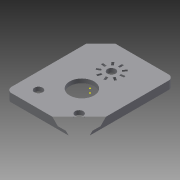
# Autodesk Inventor part: luz
Saved by Autodesk Inventor 2015 SP1 (Build 190203100, 203)
## iProperties
Created: 2015-07-05
Part Number: luz
Material: Genérico
Document SubType Name: Modeling
Designer: Javier
Density: 1 g/cm^3
Appearance: Valor por defecto
Author: Javier
Autodesk Inventor part; units mm, degrees
ref_plane "YZ Plane" through (0, 0, 0) normal (1, 0, 0) x (0, 1, 0)
ref_plane "XZ Plane" through (0, 0, 0) normal (0, 1, 0) x (-1, 0, 0)
ref_plane "XY Plane" through (0, 0, 0) normal (0, 0, 1) x (1, 0, 0)
sketch "Boceto1" plane through (0, 0, 0) normal (0, 0, 1) x (1, 0, 0)
  point P0 (0, 0)
sketch "Boceto2" plane through (0, 0, 0) normal (0, 0, 1) x (1, 0, 0)
  arc A0 (11.5, 13.5) -> (9.5, 15.5) centre (9.5, 13.5) ccw projected
  line L0 (9.5, 15.5) -> (-9.5, 15.5) projected
  arc A1 (-9.5, 15.5) -> (-11.5, 13.5) centre (-9.5, 13.5) ccw projected
  line L1 (-11.5, 13.5) -> (-11.5, -13.5) projected
  arc A2 (-11.5, -13.5) -> (-9.5, -15.5) centre (-9.5, -13.5) ccw projected
  line L2 (-9.5, -15.5) -> (9.5, -15.5) projected
  arc A3 (9.5, -15.5) -> (11.5, -13.5) centre (9.5, -13.5) ccw projected
  line L3 (11.5, -13.5) -> (11.5, 13.5) projected
  circle A4 centre (7.5, -11.5) radius 1.5 projected
  circle A5 centre (-7.5, -11.5) radius 1.5 projected
  line L4 (-4.5, 17.5) -> (-11.5, 17.5) projected
  arc A6 (-11.5, 17.5) -> (-13.5, 15.5) centre (-11.5, 15.5) ccw projected
  line L5 (-13.5, 15.5) -> (-13.5, -15.5) projected
  arc A7 (-13.5, -15.5) -> (-12.3012, -17.3325) centre (-11.5, -15.5) ccw projected
  arc A8 (-11.9943, -17.5) -> (-12.3012, -17.3325) centre (-13.1023, -19.165) ccw projected
  line L6 (11.9943, -17.5) -> (-11.9943, -17.5) projected
  arc A9 (12.3012, -17.3325) -> (11.9943, -17.5) centre (13.1023, -19.165) ccw projected
  arc A10 (12.3012, -17.3325) -> (13.5, -15.5) centre (11.5, -15.5) ccw projected
  line L7 (13.5, -15.5) -> (13.5, 15.5) projected
  arc A11 (13.5, 15.5) -> (11.5, 17.5) centre (11.5, 15.5) ccw projected
  line L8 (11.5, 17.5) -> (4.5, 17.5) projected
  line L9 (-4.5, 16.5) -> (-4.5, 17.5) projected
  line L10 (4.5, 17.5) -> (4.5, 16.5) projected
  line L11 (4.5, 16.5) -> (9.5, 16.5) projected
  arc A12 (12.5, 13.5) -> (9.5, 16.5) centre (9.5, 13.5) ccw projected
  line L12 (12.5, 13.5) -> (12.5, -13.5) projected
  arc A13 (9.5, -16.5) -> (12.5, -13.5) centre (9.5, -13.5) ccw projected
  line L13 (9.5, -16.5) -> (-9.5, -16.5) projected
  arc A14 (-12.5, -13.5) -> (-9.5, -16.5) centre (-9.5, -13.5) ccw projected
  line L14 (-12.5, -13.5) -> (-12.5, 13.5) projected
  arc A15 (-9.5, 16.5) -> (-12.5, 13.5) centre (-9.5, 13.5) ccw projected
  line L15 (-9.5, 16.5) -> (-4.5, 16.5) projected
  circle A16 centre (0, -6) radius 5.5 projected
  line L16 (-4.5, 15.5) -> (-4.5, 17.5)
  line L17 (4.5, 15.5) -> (4.5, 17.5)
  point P0 (0, 0)
  constraints: 4 end point, 2 point on line, 1 parallel, 1 vertical
extrude "Extrusión1" add sketch "Boceto2" along normal blind 2.5 contours A0 L0 L17 L11 A12 L12 A13 L13 A14 L14 A15 L15 L16 A1 L1 A2 L2 A3 L3 | L10 L8 A11 L7 A10 A9 L6 A8 A7 L5 A6 L4 L9 L15 A15 L14 A14 L13 A13 L12 A12 L11
sketch "Boceto3" plane through (0, 0, 2.5) normal (0, 0, 1) x (1, 0, 0)
  point P0 (0, 0)
lip "Labio1" kind lip height 1 width 1 edges at (11.5, 0, 0) (10.9142, -14.9142, 0) (0, -15.5, 0) (-10.9142, -14.9142, 0) (-11.5, 0, 0) (-10.9142, 14.9142, 0) (-7, 15.5, 0) (10.9142, 14.9142, 0) (7, 15.5, 0) guide face at (-12.8333, -4.5, 0)
sketch "Boceto4" plane through (0, 0, 2.5) normal (0, 0, 1) x (1, 0, 0)
  line L0 (-4.5, 17.5) -> (-11.5, 17.5) projected
  arc A0 (-11.5, 17.5) -> (-13.5, 15.5) centre (-11.5, 15.5) ccw projected
  line L1 (-13.5, 15.5) -> (-13.5, -15.5) projected
  arc A1 (-13.5, -15.5) -> (-12.3012, -17.3325) centre (-11.5, -15.5) ccw projected
  line L2 (-11.9943, -17.5) -> (11.9943, -17.5) projected
  arc A2 (12.3012, -17.3325) -> (13.5, -15.5) centre (11.5, -15.5) ccw projected
  line L3 (13.5, -15.5) -> (13.5, 15.5) projected
  arc A3 (13.5, 15.5) -> (11.5, 17.5) centre (11.5, 15.5) ccw projected
  line L4 (11.5, 17.5) -> (4.5, 17.5) projected
  line L5 (-4.5, 17.5) -> (4.5, 17.5)
  circle A4 centre (-7.5, -11.5) radius 1.5 projected
  circle A5 centre (7.5, -11.5) radius 1.5 projected
  line L6 (0, -15.5) -> (0, -3)
  circle A6 centre (0, -3) radius 4.5
  line L7 (12.3062, -17.3254) -> (11.9943, -17.5)
  arc A7 (12.3012, -17.3325) -> (11.9943, -17.5) centre (13.1023, -19.165) ccw projected
  line L8 (-12.3012, -17.3325) -> (-11.9943, -17.5)
  arc A8 (-11.9943, -17.5) -> (-12.3012, -17.3325) centre (-13.1023, -19.165) ccw projected
  dimension "d8" = 12.5
  dimension "d9" = 9
  constraints: 8 end point, 5 centre point, 1 coincident, 1 collinear, 1 vertical
  measures "d8" distance of L6.start L6.end
  measures "d9" diameter of A6
extrude "Extrusión2" add sketch "Boceto4" along normal blind 1.5 contours L5 L4 A3 L3 A2 A7 L2 A8 A1 L1 A0 L0
sketch "Boceto7" plane through (0, 0, 4) normal (0, 0, 1) x (1, 0, 0)
  circle A0 centre (0, -3) radius 4.5 projected
  circle A1 centre (7.5, -11.5) radius 1.5 projected
  circle A2 centre (-7.5, -11.5) radius 1.5 projected
  line L0 (11.5, 17.5) -> (-11.5, 17.5) projected
  arc A3 (-11.5, 17.5) -> (-13.5, 15.5) centre (-11.5, 15.5) ccw projected
  line L1 (-13.5, 15.5) -> (-13.5, -15.5) projected
  arc A4 (-13.5, -15.5) -> (-12.3012, -17.3325) centre (-11.5, -15.5) ccw projected
  line L2 (-11.9943, -17.5) -> (11.9943, -17.5) projected
  arc A5 (12.3012, -17.3325) -> (13.5, -15.5) centre (11.5, -15.5) ccw projected
  line L3 (13.5, -15.5) -> (13.5, 15.5) projected
  arc A6 (13.5, 15.5) -> (11.5, 17.5) centre (11.5, 15.5) ccw projected
  circle A7 centre (0, 7.9359) radius 1.5
  line L4 (-0.375, 12.1766) -> (0.375, 12.1766)
  line L5 (0.375, 12.1766) -> (0.375, 10.6766)
  line L6 (0.375, 10.6766) -> (-0.375, 10.6766)
  line L7 (-0.375, 10.6766) -> (-0.375, 12.1766)
  line L8 (-0.375, 12.1766) -> (0.375, 10.6766) construction
  line L9 (0.375, 12.1766) -> (-0.375, 10.6766) construction
  arc A8 (-11.9943, -17.5) -> (-12.3012, -17.3325) centre (-13.1023, -19.165) ccw projected
  arc A9 (12.3012, -17.3325) -> (11.9943, -17.5) centre (13.1023, -19.165) ccw projected
  line L10 (-3.0131, 10.9434) -> (-2.4386, 11.4255)
  line L11 (-2.4386, 11.4255) -> (-1.4744, 10.2764)
  line L12 (-1.4744, 10.2764) -> (-2.0489, 9.7943)
  line L13 (-2.0489, 9.7943) -> (-3.0131, 10.9434)
  line L14 (-3.0131, 10.9434) -> (-1.4744, 10.2764) construction
  line L15 (-2.4386, 11.4255) -> (-2.0489, 9.7943) construction
  line L16 (-4.2413, 8.303) -> (-4.1111, 9.0416)
  line L17 (-4.1111, 9.0416) -> (-2.6339, 8.7812)
  line L18 (-2.6339, 8.7812) -> (-2.7641, 8.0425)
  line L19 (-2.7641, 8.0425) -> (-4.2413, 8.303)
  line L20 (-4.2413, 8.303) -> (-2.6339, 8.7812) construction
  line L21 (-4.1111, 9.0416) -> (-2.7641, 8.0425) construction
  line L22 (-3.485, 5.4909) -> (-3.86, 6.1404)
  line L23 (-3.86, 6.1404) -> (-2.561, 6.8904)
  line L24 (-2.561, 6.8904) -> (-2.186, 6.2409)
  line L25 (-2.186, 6.2409) -> (-3.485, 5.4909)
  line L26 (-3.485, 5.4909) -> (-2.561, 6.8904) construction
  line L27 (-3.86, 6.1404) -> (-2.186, 6.2409) construction
  line L28 (-1.098, 3.8228) -> (-1.8028, 4.0793)
  line L29 (-1.8028, 4.0793) -> (-1.2897, 5.4888)
  line L30 (-1.2897, 5.4888) -> (-0.585, 5.2323)
  line L31 (-0.585, 5.2323) -> (-1.098, 3.8228)
  line L32 (-1.098, 3.8228) -> (-1.2897, 5.4888) construction
  line L33 (-1.8028, 4.0793) -> (-0.585, 5.2323) construction
  line L34 (1.8028, 4.0793) -> (1.098, 3.8228)
  line L35 (1.098, 3.8228) -> (0.585, 5.2323)
  line L36 (0.585, 5.2323) -> (1.2897, 5.4888)
  line L37 (1.2897, 5.4888) -> (1.8028, 4.0793)
  line L38 (1.8028, 4.0793) -> (0.585, 5.2323) construction
  line L39 (1.098, 3.8228) -> (1.2897, 5.4888) construction
  line L40 (3.86, 6.1404) -> (3.485, 5.4909)
  line L41 (3.485, 5.4909) -> (2.186, 6.2409)
  line L42 (2.186, 6.2409) -> (2.561, 6.8904)
  line L43 (2.561, 6.8904) -> (3.86, 6.1404)
  line L44 (3.86, 6.1404) -> (2.186, 6.2409) construction
  line L45 (3.485, 5.4909) -> (2.561, 6.8904) construction
  line L46 (4.1111, 9.0416) -> (4.2413, 8.303)
  line L47 (4.2413, 8.303) -> (2.7641, 8.0425)
  line L48 (2.7641, 8.0425) -> (2.6339, 8.7812)
  line L49 (2.6339, 8.7812) -> (4.1111, 9.0416)
  line L50 (4.1111, 9.0416) -> (2.7641, 8.0425) construction
  line L51 (4.2413, 8.303) -> (2.6339, 8.7812) construction
  line L52 (2.4386, 11.4255) -> (3.0131, 10.9434)
  line L53 (3.0131, 10.9434) -> (2.0489, 9.7943)
  line L54 (2.0489, 9.7943) -> (1.4744, 10.2764)
  line L55 (1.4744, 10.2764) -> (2.4386, 11.4255)
  line L56 (2.4386, 11.4255) -> (2.0489, 9.7943) construction
  line L57 (3.0131, 10.9434) -> (1.4744, 10.2764) construction
  point P0 (0, 11.4266)
  point P1 (-2.2437, 10.6099)
  point P2 (-3.4376, 8.5421)
  point P3 (-3.023, 6.1906)
  point P4 (-1.1939, 4.6558)
  point P5 (1.1939, 4.6558)
  point P6 (3.023, 6.1906)
  point P7 (3.4376, 8.5421)
  point P8 (2.2437, 10.6099)
  dimension "d43" = 360
  dimension "d38" = 3
  dimension "d39" = 0.75
  dimension "d47" = 360
  constraints: 108 end point, 18 midpoint, 2 parallel, 1 centre point, 1 horizontal, 1 perpendicular, 101 other
  measures "d38" diameter of A7
  measures "d39" distance of L5.end L6.end
sketch "Boceto6" plane through (0, 0, 4) normal (0, 0, 1) x (1, 0, 0)
  arc A0 (-12.3012, -17.3325) -> (-11.9943, -17.5) centre (-13.1023, -19.165) ccw projected
  arc A1 (11.9943, -17.5) -> (12.3012, -17.3325) centre (13.1023, -19.165) ccw projected
  circle A2 centre (-13.1023, -19.165) radius 2
  circle A3 centre (13.1023, -19.165) radius 2
  point P0 (0, 0)
  constraints: 2 centre point, 2 coincident, 2 concentric
extrude "Extrusión4" cut sketch "Boceto6" against normal blind 10
extrude "Extrusión5" cut sketch "Boceto7" against normal blind 10 contours A7 | L4 L5 L6 L7 | L10 L11 L12 L13 | L16 L17 L18 L19 | L22 L23 L24 L25 | L28 L29 L30 L31 | L34 L35 L36 L37 | L40 L41 L42 L43 | L46 L47 L48 L49 | L52 L53 L54 L55
